DHECelectronicschassisv2 (Autodesk Fusion 360 design; units mm, degrees)
Autodesk Fusion 360 part; units mm, degrees
sketch "Sketch1" plane through (0, 0, 0) normal (1, 0, 0) x (0, 1, 0)
  circle A0 centre (0, 0) radius 37.5
  circle A1 centre (0, 0) radius 35
  line L0 (-21.650635, 27.5) -> (-21.650635, -27.5)
  line L1 (-23.650635, 25.800145) -> (-23.650635, -25.800145)
  line L2 (0, 37.5) -> (0, -37.5)
  dimension "d1" = 75
  dimension "d2" = 2.5
  dimension "d3" = 55
  dimension "d6" = 2
  constraint coincident A0.centre A1.centre
  constraint vertical L0
  constraint vertical L1
  constraint coincident A0 L2.start
  constraint coincident A0 L2.end
  constraint vertical L2
  constraint coincident A0.centre L2
  measures "d1" diameter of A0
  measures "d2" distance of A0 A1
  measures "d6" distance of L0 L1
extrude "Extrude1" add sketch "Sketch1" against normal blind 20 contours A0 A1 L2 | A0 A1 L2 picked at (1.778935, 36.539435) picked at (-35.687243, 2.540636)
extrude "Extrude2" add sketch "Sketch1" along normal blind 120 contours A0 A1 L2 | A1 L0 L1 picked at (-35.687243, 2.540636) picked at (-22.766492, -8.972257)
sketch "Sketch2" plane through (0, 0, 0) normal (0, 1, 0) x (1, 0, 0)
  line L0 (-20, 18) -> (-5.535534, 3.535534)
  line L1 (-5.535534, -3.535534) -> (-18, -16)
  line L2 (0, -37.5) -> (0, 37.5)
  line L3 (-18, -7.514719) -> (-14.020815, -3.535534)
  line L4 (-14.020815, 3.535534) -> (-20, 9.514719)
  line L5 (-20, 37.5) -> (-20, -37.5)
  line L6 (1.75, 0) -> (22.5, 0)
  line L7 (-18, -16) -> (-18, -7.514719)
  arc A0 (-5.535534, -3.535534) -> (-5.535534, 3.535534) centre (-9.071068, 0) ccw
  arc A1 (-14.020815, -3.535534) -> (-14.020815, 3.535534) centre (-17.556349, 0) ccw
  point P0 (-2, 0)
  dimension "d9" = 2
  dimension "d10" = 6
  dimension "d12" = 6
  dimension "d13" = 2
  dimension "d14" = 5
  constraint parallel L1 L3
  constraint perpendicular L1 L4
  constraint parallel L0 L4
  constraint coincident L0.start L5
  constraint coincident P0 L6
  constraint parallel L2 L7
  constraint coincident P0 L0
  constraint coincident P0 L1
  constraint tangent L0 A0
  constraint tangent L1 A0
  constraint tangent L4 A1
  constraint tangent L3 A1
  constraint equal A0 A1
  measures "d9" distance of P0 L2
  measures "d10" distance of L1 L3
  measures "d12" distance of L0 L4
  measures "d14" radius of A0
extrude "Extrude3" cut sketch "Sketch2" along normal through all contours L0 L1 L3 L4 L5 L7 A0 A1 picked at (-15.178511, 10.350084)
sketch "Sketch3" plane through (120, 0, 0) normal (1, 0, 0) x (0, 1, 0)
  arc A0 (-23.650635, 25.800145) -> (-23.650635, -25.800145) centre (0, 0) ccw
  line L0 (-23.650635, 25.800145) -> (-23.650635, -25.800145)
  arc A1 (0, 37.5) -> (0, -37.5) centre (0, 0) ccw
  line L1 (0, -37.5) -> (0, -35)
  arc A2 (-21.650635, -27.5) -> (0, -35) centre (0, 0) ccw
  line L2 (-21.650635, -27.5) -> (-21.650635, 27.5)
  arc A3 (0, 35) -> (-21.650635, 27.5) centre (0, 0) ccw
  line L3 (0, 35) -> (0, 37.5)
  circle A4 centre (0, 0) radius 37.5
  circle A5 centre (0, 0) radius 35
  line L4 (-32.691742, -12.5) -> (-32.691742, 12.5)
  line L5 (-30.691742, 21.546855) -> (-30.691742, -21.546855)
  line L6 (-5, 37.165172) -> (-5, -37.165172)
  line L7 (5, 37.165172) -> (5, -37.165172)
  dimension "d18" = 25
  dimension "d19" = 2
  dimension "d22" = 5
  dimension "d23" = 5
  constraint coincident A0.centre A1.centre
  constraint coincident A1.start A4
  constraint coincident A3.start A5
  constraint parallel L0 L4
  constraint parallel L4 L5
  constraint parallel L6 L7
  constraint vertical L6
  measures "d19" distance of L4 L5
  measures "d22" distance of A0.centre L7
  measures "d23" distance of A0.centre L6
extrude "Extrude4" add sketch "Sketch3" along normal blind 100 contours A0 A5 L4 | A0 A1 A4 A5 L5 picked at (-33.18219, -2.536041) picked at (-34.069158, -10.871914)
extrude "Extrude5" add sketch "Sketch3" along normal blind 15 contours A1 A3 L3 A4 A5 L6 | A1 L1 A2 A4 A5 L6 | L3 A4 A5 L7 | L1 A4 A5 L7 picked at (-4.446563, 35.548829) picked at (-4.446563, -35.548829) picked at (4.446563, 35.548829) picked at (4.446563, -35.548829)
fillet "Fillet4" radius 2.5 3 edges at (-20, 34.977376, -9.514719) (-18, 35.461546, 7.514719) (-18, 32.52205, 16)
pattern_circular "C-Pattern1" count 4 over 360 about axis through (1.75, 0, 0) along (1, 0, 0) of "Extrude3", "Fillet4"
sketch "Sketch4" plane through (0, 0, 0) normal (0, 0, 1) x (1, 0, 0)
  line L0 (121, -5) -> (121, 3)
  line L1 (121, 3) -> (133, 3)
  line L2 (133, 3) -> (133, -3)
  line L3 (133, -3) -> (127, -3)
  line L4 (127, -3) -> (127, -5)
  line L5 (-14.020815, -3.535534) -> (-15.732233, -5.246952)
  line L6 (-20, 32.897568) -> (-20, -3.479185)
  arc A0 (-5.535534, 37.332961) -> (-20, 32.897568) centre (-2, 0) ccw
  spline S0 degree 3 poles (-5.535534, 37.332961) (-5.092031, 37.374962) (-4.707352, 37.419619) (-4.196849, 37.482581) (-4.071068, 37.5) (-4.071068, 37.5) knots 0.37717142 0.37717142 0.37717142 0.37717142 0.56575509 0.56575509 0.75433875 0.75433875 0.75433875 0.75433875
  arc A1 (-5.535534, 37.332961) -> (-13.732233, 35.617478) centre (-2, 0) ccw
  line L7 (-18, 36.512233) -> (-18, 36.151894)
  arc A2 (-14.020815, 37.332961) -> (-17.267767, 36.881539) centre (-10.485281, 0) ccw
  spline S1 degree 3 poles (-14.020815, 37.332961) (-13.577313, 37.374962) (-13.192633, 37.419619) (-12.682131, 37.482581) (-12.556349, 37.5) (-12.556349, 37.5) knots 1.88584893 1.88584893 1.88584893 1.88584893 2.07443259 2.07443259 2.26301626 2.26301626 2.26301626 2.26301626
  arc A3 (-14.020815, 37.332961) -> (-15.732233, 37.131112) centre (-10.485281, 0) ccw
  line L8 (-20, 37.5) -> (-20, 18)
  line L9 (-5.535534, 3.535534) -> (-20, 18)
  spline S2 degree 3 poles (-5.535534, 3.535534) (-5.092031, 3.092031) (-4.707352, 2.530295) (-4.196849, 1.298616) (-4.071068, 0.628612) (-4.071068, -0.628612) (-4.196849, -1.298616) (-4.707352, -2.530295) (-5.092031, -3.092031) (-5.535534, -3.535534) knots 0.37717142 0.37717142 0.37717142 0.37717142 0.56575509 0.56575509 0.75433875 0.75433875 0.94292242 0.94292242 1.13150609 1.13150609 1.13150609 1.13150609
  line L10 (-13.732233, -11.732233) -> (-5.535534, -3.535534)
  line L11 (-18, -8.550253) -> (-18, -9.964466)
  line L12 (-14.020815, -3.535534) -> (-17.267767, -6.782486)
  spline S3 degree 3 poles (-14.020815, -3.535534) (-13.577313, -3.092031) (-13.192633, -2.530295) (-12.682131, -1.298616) (-12.556349, -0.628612) (-12.556349, 0.628612) (-12.682131, 1.298616) (-13.192633, 2.530295) (-13.577313, 3.092031) (-14.020815, 3.535534) knots 1.88584893 1.88584893 1.88584893 1.88584893 2.07443259 2.07443259 2.26301626 2.26301626 2.45159993 2.45159993 2.64018359 2.64018359 2.64018359 2.64018359
  line L13 (-15.732233, 5.246952) -> (-14.020815, 3.535534)
  line L14 (-20, 3.479185) -> (-20, -32.897568)
  arc A4 (-20, -32.897568) -> (-5.535534, -37.332961) centre (-2, 0) ccw
  spline S4 degree 3 poles (-5.535534, -37.332961) (-5.092031, -37.374962) (-4.707352, -37.419619) (-4.196849, -37.482581) (-4.071068, -37.5) (-4.071068, -37.5) knots 0.37717142 0.37717142 0.37717142 0.37717142 0.56575509 0.56575509 0.75433875 0.75433875 0.75433875 0.75433875
  arc A5 (-13.732233, -35.617478) -> (-5.535534, -37.332961) centre (-2, 0) ccw
  line L15 (-18, -36.151894) -> (-18, -36.512233)
  arc A6 (-17.267767, -36.881539) -> (-14.020815, -37.332961) centre (-10.485281, 0) ccw
  spline S5 degree 3 poles (-14.020815, -37.332961) (-13.577313, -37.374962) (-13.192633, -37.419619) (-12.682131, -37.482581) (-12.556349, -37.5) (-12.556349, -37.5) knots 1.88584893 1.88584893 1.88584893 1.88584893 2.07443259 2.07443259 2.26301626 2.26301626 2.26301626 2.26301626
  arc A7 (-15.732233, -37.131112) -> (-14.020815, -37.332961) centre (-10.485281, 0) ccw
  line L16 (-20, -18) -> (-20, -37.5)
  line L17 (-20, -18) -> (-5.535534, -3.535534)
  spline S6 degree 3 poles (-5.535534, -3.535534) (-5.092031, -3.092031) (-4.707352, -2.530295) (-4.196849, -1.298616) (-4.071068, -0.628612) (-4.071068, 0.628612) (-4.196849, 1.298616) (-4.707352, 2.530295) (-5.092031, 3.092031) (-5.535534, 3.535534) knots 0.37717142 0.37717142 0.37717142 0.37717142 0.56575509 0.56575509 0.75433875 0.75433875 0.94292242 0.94292242 1.13150609 1.13150609 1.13150609 1.13150609
  line L18 (-5.535534, 3.535534) -> (-13.732233, 11.732233)
  line L19 (-18, 9.964466) -> (-18, 8.550253)
  line L20 (-17.267767, 6.782486) -> (-14.020815, 3.535534)
  spline S7 degree 3 poles (-14.020815, 3.535534) (-13.577313, 3.092031) (-13.192633, 2.530295) (-12.682131, 1.298616) (-12.556349, 0.628612) (-12.556349, -0.628612) (-12.682131, -1.298616) (-13.192633, -2.530295) (-13.577313, -3.092031) (-14.020815, -3.535534) knots 1.88584893 1.88584893 1.88584893 1.88584893 2.07443259 2.07443259 2.26301626 2.26301626 2.45159993 2.45159993 2.64018359 2.64018359 2.64018359 2.64018359
  line L21 (0, 0) -> (0, 37.5)
  line L22 (0, 0) -> (120, 0)
  line L23 (120, 0) -> (120, 5)
  line L24 (120, 5) -> (135, 5)
  line L25 (135, -5) -> (135, 5)
  line L26 (135, -5) -> (120, -5)
  line L27 (120, -30.691742) -> (120, -5)
  line L28 (120, -30.691742) -> (220, -30.691742)
  line L29 (220, -37.5) -> (220, -30.691742)
  line L30 (220, -30.691742) -> (120, -30.691742)
  line L31 (120, -30.691742) -> (120, -5)
  line L32 (120, -5) -> (135, -5)
  line L33 (135, -5) -> (135, 5)
  line L34 (135, 5) -> (120, 5)
  line L35 (120, 0) -> (120, 5)
  line L36 (120, 0) -> (0, 0)
  spline S8 degree 3 poles (-20, 37.338255) (-20, 37.308918) (-19.936932, 37.273238) (-19.68092, 37.199746) (-19.487989, 37.162156) (-19.043908, 37.099555) (-18.763574, 37.070336) (-18.148641, 37.030566) (-17.814016, 37.020256) (-17.185984, 37.020256) (-16.851359, 37.030566) (-16.236426, 37.070336) (-15.956092, 37.099555) (-15.73396, 37.130868) (-15.733096, 37.13099) (-15.732233, 37.131112) knots 0.37712173 0.37712173 0.37712173 0.37712173 0.47198416 0.47198416 0.56684658 0.56684658 0.66105142 0.66105142 0.75525626 0.75525626 0.8494611 0.8494611 0.94366594 0.94366594 0.94403377 0.94403377 0.94403377 0.94403377
  spline S9 degree 3 poles (-18, 36.151894) (-18, 36.064515) (-17.936188, 35.966567) (-17.676304, 35.777332) (-17.480233, 35.686263) (-17.033546, 35.541557) (-16.756749, 35.477172) (-16.146883, 35.390176) (-15.813717, 35.367882) (-15.186283, 35.367882) (-14.853117, 35.390176) (-14.243251, 35.477172) (-13.966454, 35.541557) (-13.742971, 35.613955) (-13.737595, 35.615712) (-13.732233, 35.617478) knots 0.38229389 0.38229389 0.38229389 0.38229389 0.48094505 0.48094505 0.57959622 0.57959622 0.67371142 0.67371142 0.76782663 0.76782663 0.86194184 0.86194184 0.95605704 0.95605704 0.95838506 0.95838506 0.95838506 0.95838506
  spline S10 degree 3 poles (-17.267767, 36.881539) (-17.490895, 36.840485) (-17.68265, 36.786532) (-17.937795, 36.659201) (-18, 36.585418) (-18, 36.512233) knots 0.18895467 0.18895467 0.18895467 0.18895467 0.28431905 0.28431905 0.38061126 0.38061126 0.38061126 0.38061126
  spline S11 degree 3 poles (-20, -3.479185) (-20, -3.794029) (-19.936932, -4.129428) (-19.68092, -4.746086) (-19.487989, -5.027377) (-19.043908, -5.47016) (-18.763574, -5.66187) (-18.148641, -5.916396) (-17.814016, -5.979185) (-17.185984, -5.979185) (-16.851359, -5.916396) (-16.236426, -5.66187) (-15.956092, -5.47016) (-15.73396, -5.248677) (-15.733096, -5.247815) (-15.732233, -5.246952) knots 0.37712173 0.37712173 0.37712173 0.37712173 0.47198416 0.47198416 0.56684658 0.56684658 0.66105142 0.66105142 0.75525626 0.75525626 0.8494611 0.8494611 0.94366594 0.94366594 0.94403377 0.94403377 0.94403377 0.94403377
  spline S12 degree 3 poles (-18, -9.964466) (-18, -10.281482) (-17.936188, -10.61892) (-17.676304, -11.240015) (-17.480233, -11.523738) (-17.033546, -11.962381) (-16.756749, -12.150634) (-16.146883, -12.401737) (-15.813717, -12.464466) (-15.186283, -12.464466) (-14.853117, -12.401737) (-14.243251, -12.150634) (-13.966454, -11.962381) (-13.742971, -11.742923) (-13.737595, -11.737592) (-13.732233, -11.732233) knots 0.38229389 0.38229389 0.38229389 0.38229389 0.48094505 0.48094505 0.57959622 0.57959622 0.67371142 0.67371142 0.76782663 0.76782663 0.86194184 0.86194184 0.95605704 0.95605704 0.95838506 0.95838506 0.95838506 0.95838506
  spline S13 degree 3 poles (-17.267767, -6.782486) (-17.490895, -7.005712) (-17.68265, -7.286905) (-17.937795, -7.902709) (-18, -8.237733) (-18, -8.550253) knots 0.18895467 0.18895467 0.18895467 0.18895467 0.28431905 0.28431905 0.38061126 0.38061126 0.38061126 0.38061126
  spline S14 degree 3 poles (-20, 3.479185) (-20, 3.794029) (-19.936932, 4.129428) (-19.68092, 4.746086) (-19.487989, 5.027377) (-19.043908, 5.47016) (-18.763574, 5.66187) (-18.148641, 5.916396) (-17.814016, 5.979185) (-17.185984, 5.979185) (-16.851359, 5.916396) (-16.236426, 5.66187) (-15.956092, 5.47016) (-15.73396, 5.248677) (-15.733096, 5.247815) (-15.732233, 5.246952) knots 0.37712173 0.37712173 0.37712173 0.37712173 0.47198416 0.47198416 0.56684658 0.56684658 0.66105142 0.66105142 0.75525626 0.75525626 0.8494611 0.8494611 0.94366594 0.94366594 0.94403377 0.94403377 0.94403377 0.94403377
  spline S15 degree 3 poles (-18, -36.151894) (-18, -36.064515) (-17.936188, -35.966567) (-17.676304, -35.777332) (-17.480233, -35.686263) (-17.033546, -35.541557) (-16.756749, -35.477172) (-16.146883, -35.390176) (-15.813717, -35.367882) (-15.186283, -35.367882) (-14.853117, -35.390176) (-14.243251, -35.477172) (-13.966454, -35.541557) (-13.742971, -35.613955) (-13.737595, -35.615712) (-13.732233, -35.617478) knots 0.38229389 0.38229389 0.38229389 0.38229389 0.48094505 0.48094505 0.57959622 0.57959622 0.67371142 0.67371142 0.76782663 0.76782663 0.86194184 0.86194184 0.95605704 0.95605704 0.95838506 0.95838506 0.95838506 0.95838506
  spline S16 degree 3 poles (-17.267767, -36.881539) (-17.490895, -36.840485) (-17.68265, -36.786532) (-17.937795, -36.659201) (-18, -36.585418) (-18, -36.512233) knots 0.18895467 0.18895467 0.18895467 0.18895467 0.28431905 0.28431905 0.38061126 0.38061126 0.38061126 0.38061126
  spline S17 degree 3 poles (-20, -37.338255) (-20, -37.308918) (-19.936932, -37.273238) (-19.68092, -37.199746) (-19.487989, -37.162156) (-19.043908, -37.099555) (-18.763574, -37.070336) (-18.148641, -37.030566) (-17.814016, -37.020256) (-17.185984, -37.020256) (-16.851359, -37.030566) (-16.236426, -37.070336) (-15.956092, -37.099555) (-15.73396, -37.130868) (-15.733096, -37.13099) (-15.732233, -37.131112) knots 0.37712173 0.37712173 0.37712173 0.37712173 0.47198416 0.47198416 0.56684658 0.56684658 0.66105142 0.66105142 0.75525626 0.75525626 0.8494611 0.8494611 0.94366594 0.94366594 0.94403377 0.94403377 0.94403377 0.94403377
  spline S18 degree 3 poles (-18, 9.964466) (-18, 10.281482) (-17.936188, 10.61892) (-17.676304, 11.240015) (-17.480233, 11.523738) (-17.033546, 11.962381) (-16.756749, 12.150634) (-16.146883, 12.401737) (-15.813717, 12.464466) (-15.186283, 12.464466) (-14.853117, 12.401737) (-14.243251, 12.150634) (-13.966454, 11.962381) (-13.742971, 11.742923) (-13.737595, 11.737592) (-13.732233, 11.732233) knots 0.38229389 0.38229389 0.38229389 0.38229389 0.48094505 0.48094505 0.57959622 0.57959622 0.67371142 0.67371142 0.76782663 0.76782663 0.86194184 0.86194184 0.95605704 0.95605704 0.95838506 0.95838506 0.95838506 0.95838506
  spline S19 degree 3 poles (-17.267767, 6.782486) (-17.490895, 7.005712) (-17.68265, 7.286905) (-17.937795, 7.902709) (-18, 8.237733) (-18, 8.550253) knots 0.18895467 0.18895467 0.18895467 0.18895467 0.28431905 0.28431905 0.38061126 0.38061126 0.38061126 0.38061126
  dimension "d26" = 6
  dimension "d27" = 6
  dimension "d28" = 6
  dimension "d29" = 2
  dimension "d30" = 2
  constraint vertical L0
  constraint perpendicular L0 L1
  constraint perpendicular L1 L2
  constraint perpendicular L2 L3
  constraint perpendicular L3 L4
  measures "d26" distance of L0 L4
  measures "d27" distance of L1 L3
  measures "d28" distance of L2.end L3.end
  measures "d29" distance of L2 L25
  measures "d30" distance of L1 L24
extrude "Extrude6" cut sketch "Sketch4" along normal through all and the other way through all contours L0 L1 L2 L3 L4 L26 L32 picked at (127, 1)
chamfer "Chamfer2" distance 5 angle 45 2 edges at (120, 0, 36.25) (120, 0, -36.25)
chamfer "Chamfer3" distance 1 angle 45 2 edges at (120, -5, 35.903094) (120, -5, -35.903094)
fillet "Fillet1" radius 10 2 edges at (0, 0, 36.25) (0, 0, -36.25)
fillet "Fillet2" radius 5 2 edges at (120, -30.691742, 19.184982) (120, -30.691742, -19.184982)
fillet "Fillet3" radius 2.5 12 edges at (135, 5, 35.903094) (135, -5, 35.903094) (120, 5, 35.903094) (120, 5, -35.903094) (135, 5, -35.903094) (135, -5, -35.903094) (133, 3, -36.125499) (121, 3, -36.125499) (133, -3, -36.125499) (133, 3, 36.125499) (121, 3, 36.125499) (133, -3, 36.125499)
sketch "Sketch5" plane through (0, -21.650635, 0) normal (0, 1, 0) x (-1, 0, 0)
  line L0 (0, -27.5) -> (0, 27.5)
  line L1 (0, 27.5) -> (-120, 27.5)
  line L2 (-120, 27.5) -> (-120, -27.5)
  line L3 (-120, -27.5) -> (0, -27.5)
  line L4 (-120, 17.5) -> (-102.387321, 17.5)
  line L5 (-99.571068, 7.5) -> (-120, 7.5)
  line L6 (-100, 0) -> (-82.32233, 17.67767)
  line L7 (-82.32233, 17.67767) -> (-64.644661, 0)
  line L8 (-64.644661, 0) -> (-82.32233, -17.67767)
  line L9 (-82.32233, -17.67767) -> (-100, 0)
  line L10 (-55.355339, 0) -> (-37.67767, 17.67767)
  line L11 (-37.67767, 17.67767) -> (-20, 0)
  line L12 (-20, 0) -> (-37.67767, -17.67767)
  line L13 (-37.67767, -17.67767) -> (-55.355339, 0)
  line L14 (-1.75, 0) -> (-22.5, 0)
  line L15 (-85.073593, 27.5) -> (-60, 2.426407)
  line L16 (-60, 2.426407) -> (-34.926407, 27.5)
  line L17 (-34.926407, 27.5) -> (-85.073593, 27.5)
  line L18 (-99.571068, 7.5) -> (-89.571068, 17.5)
  line L19 (-89.571068, 17.5) -> (-102.387321, 17.5)
  line L20 (-60, 2.426407) -> (-60, 27.5) construction
  line L21 (0, 17.5) -> (-17.612679, 17.5)
  line L22 (-30.428932, 17.5) -> (-17.612679, 17.5)
  line L23 (-20.428932, 7.5) -> (-30.428932, 17.5)
  line L24 (-20.428932, 7.5) -> (0, 7.5)
  line L25 (-99.571068, -7.5) -> (-120, -7.5)
  line L26 (-99.571068, -7.5) -> (-89.571068, -17.5)
  line L27 (-89.571068, -17.5) -> (-102.387321, -17.5)
  line L28 (-85.073593, -27.5) -> (-60, -2.426407)
  line L29 (-34.926407, -27.5) -> (-85.073593, -27.5)
  line L30 (-60, -2.426407) -> (-34.926407, -27.5)
  line L31 (0, -17.5) -> (-17.612679, -17.5)
  line L32 (-30.428932, -17.5) -> (-17.612679, -17.5)
  line L33 (-20.428932, -7.5) -> (-30.428932, -17.5)
  line L34 (-20.428932, -7.5) -> (0, -7.5)
  line L35 (-102.387321, -17.5) -> (-120, -17.5)
  dimension "d43" = 25
  dimension "d44" = 20
  dimension "d45" = 20
  dimension "d46" = 5
  dimension "d47" = 5
  dimension "d48" = 10
  dimension "d49" = 10
  dimension "d50" = 5
  constraint coincident L2 L4.start
  constraint perpendicular L2 L4
  constraint coincident L2 L5.end
  constraint perpendicular L2 L5
  constraint perpendicular L6 L7
  constraint parallel L6 L8
  constraint parallel L7 L9
  constraint perpendicular L10 L11
  constraint parallel L10 L12
  constraint parallel L11 L13
  constraint perpendicular L9 L10
  constraint equal L10 L13
  constraint equal L7 L10
  constraint equal L7 L8
  constraint coincident L6.start L14
  constraint coincident L11.end L14
  constraint perpendicular L8 L15
  constraint perpendicular L7 L16
  constraint horizontal L17
  constraint parallel L6 L18
  constraint parallel L4 L19
  constraint coincident L1.end L17
  constraint midpoint L17 L20.end
  constraint symmetric L4.start L20 L21.start
  constraint symmetric L5.end L20 L24.end
  constraint symmetric L5.end L14 L25.end
  constraint symmetric L14 L21.start L31.start
  constraint symmetric L14 L24.end L34.end
  constraint coincident L2 L35.end
  constraint perpendicular L2 L35
  measures "d44" distance of L2 L6.start
  measures "d45" distance of origin L11.end
  measures "d46" distance of L7 L15
  measures "d47" distance of L10 L16
  measures "d48" distance of L4 L5
  measures "d49" distance of L1 L4
  measures "d50" distance of L6 L18
extrude "Extrude7" cut sketch "Sketch5" against normal through all contours L0 L31 L32 L33 L34 | L3 L28 L29 L30 | L0 L21 L22 L23 L24 | L2 L25 L26 L27 L35 | L1 L15 L16 L17 | L2 L4 L5 L18 L19 | L6 L7 L8 L9 | L10 L11 L12 L13 picked at (-12.680537, -10.833333) picked at (-60, -19.142136) picked at (-12.680537, 10.833333) picked at (-107.319463, -10.833333) picked at (-60, 19.142136) picked at (-107.319463, 10.833333) picked at (-76.429774, 0) picked at (-31.785113, 0)
sketch "Sketch6" plane through (0, -32.691742, 0) normal (0, 1, 0) x (-1, 0, 0)
  line L0 (-120, -12.5) -> (-120, 12.5)
  line L1 (-120, 12.5) -> (-220, 12.5)
  line L2 (-220, 12.5) -> (-220, -12.5)
  line L3 (-220, -12.5) -> (-120, -12.5)
  line L4 (-210, 0) -> (-197.5, 12.5)
  line L5 (-197.5, 12.5) -> (-185, 0)
  line L6 (-185, 0) -> (-197.5, -12.5)
  line L7 (-197.5, -12.5) -> (-210, 0)
  line L8 (-180, 0) -> (-167.5, 12.5)
  line L9 (-167.5, 12.5) -> (-155, 0)
  line L10 (-155, 0) -> (-167.5, -12.5)
  line L11 (-167.5, -12.5) -> (-180, 0)
  line L12 (-150, 0) -> (-137.5, 12.5)
  line L13 (-137.5, 12.5) -> (-125, 0)
  line L14 (-125, 0) -> (-137.5, -12.5)
  line L15 (-137.5, -12.5) -> (-150, 0)
  line L16 (-1.75, 0) -> (-22.5, 0)
  line L17 (-193.257359, 12.5) -> (-182.5, 1.742641)
  line L18 (-182.5, 1.742641) -> (-171.742641, 12.5)
  line L19 (-220, 5) -> (-209.242641, 5)
  line L20 (-209.242641, 5) -> (-201.742641, 12.5)
  line L21 (-220, 5) -> (-220, 12.5)
  line L22 (-220, 12.5) -> (-120, 12.5)
  line L23 (-167.5, 12.5) -> (-167.5, -12.5) construction
  line L24 (-152.5, 1.742641) -> (-163.257359, 12.5)
  line L25 (-141.742641, 12.5) -> (-152.5, 1.742641)
  line L26 (-2.5, 0) -> (-20, 0)
  line L27 (-220, -5) -> (-209.242641, -5)
  line L28 (-209.242641, -5) -> (-201.742641, -12.5)
  line L29 (-220, -5) -> (-220, -12.5)
  line L30 (-220, -12.5) -> (-120, -12.5)
  line L31 (-193.257359, -12.5) -> (-182.5, -1.742641)
  line L32 (-182.5, -1.742641) -> (-171.742641, -12.5)
  line L33 (-152.5, -1.742641) -> (-163.257359, -12.5)
  line L34 (-141.742641, -12.5) -> (-152.5, -1.742641)
  dimension "d52" = 5
  dimension "d53" = 5
  dimension "d54" = 5
  dimension "d55" = 25
  dimension "d56" = 3
  dimension "d57" = 3
  dimension "d58" = 3
  dimension "d59" = 5
  constraint perpendicular L4 L5
  constraint parallel L4 L6
  constraint parallel L5 L7
  constraint perpendicular L8 L9
  constraint parallel L8 L10
  constraint parallel L9 L11
  constraint perpendicular L7 L8
  constraint perpendicular L12 L13
  constraint parallel L12 L14
  constraint parallel L13 L15
  constraint perpendicular L9 L12
  constraint equal L4 L5
  constraint equal L8 L9
  constraint equal L12 L13
  constraint equal L9 L12
  constraint equal L5 L8
  constraint coincident L13.end L16
  constraint coincident L12.start L16
  constraint coincident L9.end L16
  constraint coincident L5.end L16
  constraint perpendicular L17 L18
  constraint coincident L2 L19.start
  constraint perpendicular L2 L19
  constraint perpendicular L5 L20
  constraint coincident L1.end L2.start
  constraint coincident L0.end L1.start
  constraint parallel L5 L17
  constraint symmetric L19.start L26 L27.start
  constraint symmetric L1.end L26 L2.end
  constraint symmetric L0.end L26 L0.start
  measures "d52" distance of L5.end L8.start
  measures "d53" distance of L9.end L12.start
  measures "d54" distance of L0 L13.end
  measures "d55" distance of L12.end L14.end
  measures "d56" distance of L5 L17
  measures "d57" distance of L8 L18
  measures "d58" distance of L4 L20
  measures "d59" distance of L4.start L19
extrude "Extrude8" cut sketch "Sketch6" against normal through all contours L12 L13 L14 L15 | L3 L30 L33 L34 | L1 L22 L24 L25 | L8 L9 L10 L11 | L3 L30 L31 L32 | L1 L17 L18 L22 | L4 L5 L6 L7 | L2 L3 L27 L28 L29 L30 | L1 L2 L19 L20 L21 L22 picked at (-137.5, -4.166667) picked at (-152.5, -8.914214) picked at (-152.5, 8.914214) picked at (-171.666667, 0) picked at (-182.5, -8.914214) picked at (-182.5, 8.914214) picked at (-193.333333, 0) picked at (-210.328427, -10) picked at (-210.328427, 10)
